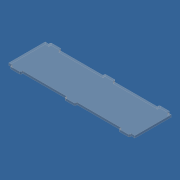
# Autodesk Inventor part: P1704_002
Saved by Autodesk Inventor 2015 (Build 190159000, 159)
## iProperties
Created: 2017-02-08
Part Number: P1704_002
Project: Polymanette chevalier
Material: Plastique PMMA
Description: Paroi arrière
Document SubType Name: Modeling
Designer: Alexandre.PICOTTE
Authority: 180x58x3
Density: 1.188 g/cm^3
Appearance: Transparent - Clair
Mass: 34.2747 g
Surface Area: 207.616 cm^2
Volume: 28.8508 cm^3
Material number: ---
Author: Boris.GAUDARD
Autodesk Inventor part; units mm, degrees
ref_plane "Plan YZ" through (0, 0, 0) normal (1, 0, 0) x (0, 1, 0)
ref_plane "Plan XZ" through (0, 0, 0) normal (0, 1, 0) x (-1, 0, 0)
ref_plane "Plan XY" through (0, 0, 0) normal (0, 0, 1) x (1, 0, 0)
sketch "Esquisse7" plane through (0, 0, 0) normal (0, 0, 1) x (1, 0, 0)
  line L0 (-90, -26) -> (-90, 26)
  line L1 (-90, 26) -> (-85, 26)
  line L2 (-85, 26) -> (-85, 29)
  line L3 (-85, 29) -> (-70, 29)
  line L4 (-70, 29) -> (-70, 26)
  line L5 (-70, 26) -> (-7.5, 26)
  line L6 (-7.5, 26) -> (-7.5, 29)
  line L7 (-7.5, 29) -> (7.5, 29)
  line L8 (7.5, 29) -> (7.5, 26)
  line L9 (7.5, 26) -> (70, 26)
  line L10 (70, 26) -> (70, 29)
  line L11 (70, 29) -> (85, 29)
  line L12 (85, 29) -> (85, 26)
  line L13 (85, 26) -> (90, 26)
  line L14 (90, 26) -> (90, -26)
  line L15 (90, -26) -> (85, -26)
  line L16 (85, -26) -> (85, -29)
  line L17 (85, -29) -> (70, -29)
  line L18 (70, -29) -> (70, -26)
  line L19 (7.5, -26) -> (7.5, -29)
  line L20 (7.5, -26) -> (70, -26)
  line L21 (7.5, -29) -> (-7.5, -29)
  line L22 (-7.5, -29) -> (-7.5, -26)
  line L23 (-7.5, -26) -> (-70, -26)
  line L24 (-70, -26) -> (-70, -29)
  line L25 (-70, -29) -> (-85, -29)
  line L26 (-85, -29) -> (-85, -26)
  line L27 (-85, -26) -> (-90, -26)
  line L28 (0, -40.6) -> (0, 40.6) construction
  line L29 (-126, 0) -> (126, 0) construction
  dimension "d33" = 52
  dimension "d34" = 15
  dimension "d35" = 3
  dimension "d36" = 5
  dimension "d37" = 77.5
  constraints: 56 end point, 24 point on line, 15 perpendicular, 7 equal length, 2 horizontal, 1 vertical, 3 other
  measures "d33" distance of L0.start L0.end
  measures "d34" distance of L2.end L3.end
  measures "d35" distance of L1.end L2.end
  measures "d36" distance of L0.end L1.end
  measures "d37" distance between parallel lines of L6 L2
extrude "Extrusion2" add sketch "Esquisse7" against normal blind 3
sketch "Esquisse8" plane through (0, 0, 0) normal (0, 0, 1) x (1, 0, 0)
  point P0 (0, 0)
  point P1 (7.5, 26)
  point P2 (-7.5, 26)
  point P3 (-85, 26)
  point P4 (-70, 26)
  point P5 (-85, -26)
  point P6 (-70, -26)
  point P7 (-7.5, -26)
  point P8 (7.5, -26)
  point P9 (70, -26)
  point P10 (85, -26)
  point P11 (70, 26)
  point P12 (85, 26)
  point P13 (85, 26)
  point P14 (70, -26)
  point P15 (85, 26)
  constraints: 3 coincident
hole "Perçage2" at (7.5, 26, 0) at (-7.5, 26, 0) at (-85, 26, 0) at (-70, 26, 0) at (-85, -26, 0) at (-70, -26, 0) at (-7.5, -26, 0) at (7.5, -26, 0) at (70, -26, 0) at (85, -26, 0) at (70, 26, 0) at (85, 26, 0) direction (0, 0, -1) diameter 1 end through all
chamfer "Chanfrein3" distance 1 angle 45 12 edges at (-85, -29, -1.5) (-70, -29, -1.5) (-85, 29, -1.5) (-70, 29, -1.5) (-7.5, 29, -1.5) (7.5, 29, -1.5) (70, 29, -1.5) (85, 29, -1.5) (70, -29, -1.5) (85, -29, -1.5) (-7.5, -29, -1.5) (7.5, -29, -1.5)
